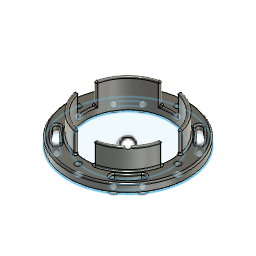
plunger holder v1 (Autodesk Fusion 360 design; units mm, degrees)
Autodesk Fusion 360 part; units mm, degrees
sketch "Sketch1" plane through (0, 0, 0) normal (0, 0, 1) x (1, 0, 0)
  circle A0 centre (-41.909966, 0.053051) radius 2.55
  circle A1 centre (41.91, 0) radius 2.55
  circle A2 centre (0, -41.910001) radius 2.55
  circle A3 centre (0, 41.910001) radius 2.55
  arc A4 (-25.400001, 38.100001) -> (-38.100001, 25.400001) centre (0, 0) ccw
  arc A5 (-38.100001, -25.400001) -> (-25.400001, -38.100001) centre (0, 0) ccw
  arc A6 (25.400001, -38.100001) -> (38.100001, -25.400001) centre (-1.334562, 1.334562) ccw
  arc A7 (38.100001, 25.400001) -> (25.400001, 38.100001) centre (-1.334562, -1.334562) ccw
  arc A8 (-22.582124, 33.873186) -> (-33.873186, 22.582124) centre (0, 0) ccw
  arc A9 (33.873186, 22.582124) -> (22.582124, 33.873186) centre (0, 0) ccw
  arc A10 (22.582124, -33.873186) -> (33.873186, -22.582124) centre (0, 0) ccw
  arc A11 (-33.873186, -22.582124) -> (-22.582124, -33.873186) centre (0, 0) ccw
  arc A12 (-33.873186, -22.582124) -> (-38.100001, -25.400001) centre (-35.986593, -23.991062) ccw
  arc A13 (-38.100001, 25.400001) -> (-33.873186, 22.582124) centre (-35.986593, 23.991062) ccw
  arc A14 (-22.582124, 33.873186) -> (-25.400001, 38.100001) centre (-23.991062, 35.986593) ccw
  arc A15 (25.400001, 38.100001) -> (22.582124, 33.873186) centre (23.991062, 35.986593) ccw
  arc A16 (33.873186, 22.582124) -> (38.100001, 25.400001) centre (35.986593, 23.991062) ccw
  arc A17 (38.100001, -25.400001) -> (33.873186, -22.582124) centre (35.99754, -23.974643) ccw
  arc A18 (22.582124, -33.873186) -> (25.400001, -38.100001) centre (23.974643, -35.99754) ccw
  arc A19 (-25.400001, -38.100001) -> (-22.582124, -33.873186) centre (-23.991062, -35.986593) ccw
  circle A20 centre (0, 0) radius 34.925
  circle A21 centre (0, 0) radius 50.165
  dimension "d4" = 5.1
  dimension "d5" = 5.1
  dimension "d6" = 5.1
  dimension "d7" = 5.1
  dimension "d24" = 69.85
  dimension "d25" = 100.33
  constraint tangent A5 A12
  constraint tangent A4 A13
  constraint tangent A8 A14
  constraint tangent A9 A15
  constraint tangent A9 A16
  constraint tangent A6 A17
  constraint tangent A6 A18
  constraint tangent A5 A19
  constraint concentric A10 A20
  measures "d4" diameter of A0
  measures "d5" diameter of A1
  measures "d6" diameter of A2
  measures "d7" diameter of A3
  measures "d24" diameter of A20
  measures "d25" diameter of A21
extrude "Extrude5" add sketch "Sketch1" along normal blind 7.62 contours A21 picked at (-41.009698, -9.190179)
sketch "Sketch3" plane through (0, 0, 7.62) normal (0, 0, 1) x (-1, 0, 0)
  arc A0 (-33.873186, -22.582124) -> (-38.100001, -25.400001) centre (-35.986593, -23.991062) ccw
  arc A1 (-33.873186, -22.582124) -> (-22.582124, -33.873186) centre (0, 0) ccw
  arc A2 (-25.400001, -38.100001) -> (-22.582124, -33.873186) centre (-23.991062, -35.986593) ccw
  arc A3 (-38.100001, -25.400001) -> (-25.400001, -38.100001) centre (1.334562, 1.334562) ccw
  circle A4 centre (-41.91, 0) radius 2.55
  circle A5 centre (0, 41.910001) radius 2.55
  arc A6 (-22.582124, 33.873186) -> (-25.400001, 38.100001) centre (-23.974643, 35.99754) ccw
  arc A7 (-22.582124, 33.873186) -> (-33.873186, 22.582124) centre (0, 0) ccw
  arc A8 (-38.100001, 25.400001) -> (-33.873186, 22.582124) centre (-35.99754, 23.974643) ccw
  arc A9 (-25.400001, 38.100001) -> (-38.100001, 25.400001) centre (1.334562, -1.334562) ccw
  arc A10 (22.582124, -33.873186) -> (25.400001, -38.100001) centre (23.991062, -35.986593) ccw
  arc A11 (22.582124, -33.873186) -> (33.873186, -22.582124) centre (0, 0) ccw
  arc A12 (38.100001, -25.400001) -> (33.873186, -22.582124) centre (35.986593, -23.991062) ccw
  arc A13 (25.400001, -38.100001) -> (38.100001, -25.400001) centre (0, 0) ccw
  circle A14 centre (41.909966, -0.053051) radius 2.55
  circle A15 centre (0, -41.910001) radius 2.55
  arc A16 (33.873186, 22.582124) -> (38.100001, 25.400001) centre (35.986593, 23.991062) ccw
  arc A17 (33.873186, 22.582124) -> (22.582124, 33.873186) centre (0, 0) ccw
  arc A18 (25.400001, 38.100001) -> (22.582124, 33.873186) centre (23.991062, 35.986593) ccw
  arc A19 (38.100001, 25.400001) -> (25.400001, 38.100001) centre (0, 0) ccw
  circle A20 centre (0, 0) radius 34.925
  circle A21 centre (0, 0) radius 50.165
  arc A22 (-8.470557, 33.882227) -> (-33.882227, 8.470557) centre (0, 0) ccw
  arc A23 (-9.086597, 36.346388) -> (-36.346388, 9.086597) centre (0, 0) ccw
  arc A24 (33.882227, 8.470557) -> (8.470557, 33.882227) centre (0, 0) ccw
  arc A25 (36.346388, 9.086597) -> (9.086597, 36.346388) centre (0, 0) ccw
  arc A26 (8.470557, -33.882227) -> (33.882227, -8.470557) centre (0, 0) ccw
  arc A27 (9.086597, -36.346388) -> (36.346388, -9.086597) centre (0, 0) ccw
  arc A28 (-33.882227, -8.470557) -> (-8.470557, -33.882227) centre (0, 0) ccw
  arc A29 (-36.346388, -9.086597) -> (-9.086597, -36.346388) centre (0, 0) ccw
  arc A30 (33.882227, 8.470557) -> (36.346388, 9.086597) centre (35.114308, 8.778577) ccw
  arc A31 (9.086597, 36.346388) -> (8.470557, 33.882227) centre (8.778577, 35.114308) ccw
  arc A32 (-8.470557, 33.882227) -> (-9.086597, 36.346388) centre (-8.778577, 35.114308) ccw
  arc A33 (-36.346388, 9.086597) -> (-33.882227, 8.470557) centre (-35.114308, 8.778577) ccw
  arc A34 (-33.882227, -8.470557) -> (-36.346388, -9.086597) centre (-35.114308, -8.778577) ccw
  arc A35 (-9.086597, -36.346388) -> (-8.470557, -33.882227) centre (-8.778577, -35.114308) ccw
  arc A36 (8.470557, -33.882227) -> (9.086597, -36.346388) centre (8.778577, -35.114308) ccw
  arc A37 (36.346388, -9.086597) -> (33.882227, -8.470557) centre (35.114308, -8.778577) ccw
  constraint tangent A25 A30
  constraint tangent A24 A31
  constraint tangent A23 A32
  constraint tangent A22 A33
  constraint tangent A28 A34
  constraint tangent A28 A35
  constraint tangent A26 A36
  constraint tangent A27 A37
extrude "Extrude6" add sketch "Sketch3" along normal blind 17.78 contours A20 A24 A25 A30 A31 | A20 A26 A27 A36 A37 | A20 A22 A23 A32 A33 | A20 A28 A29 A34 A35 picked at (35.006625, 10.485532) picked at (34.523393, -11.981049) picked at (-16.52197, 32.59501) picked at (-11.981049, -34.523393)
fillet "Fillet1" radius 1.27 16 edges at (26.491755, -26.491755, 25.4) (35.422328, -7.546496, 25.4) (24.695704, -24.695704, 25.4) (7.546496, -35.422328, 25.4) (-26.491755, -26.491755, 25.4) (-7.546496, -35.422328, 25.4) (-24.695704, -24.695704, 25.4) (-35.422328, -7.546496, 25.4) (26.491755, 26.491755, 25.4) (7.546496, 35.422328, 25.4) (24.695704, 24.695704, 25.4) (35.422328, 7.546496, 25.4) (-24.695704, 24.695704, 25.4) (-7.546496, 35.422328, 25.4) (-26.491755, 26.491755, 25.4) (-35.422328, 7.546496, 25.4)
fillet "Fillet4" radius 1.27 4 edges at (0, 34.925, 7.62) (34.925, 0, 7.62) (-34.925, 0, 7.62) (0, -34.925, 7.62)
fillet "Fillet5" radius 1.27 20 edges at (7.752154, 34.366403, 7.175515) (8.115639, 36.19755, 7.62) (26.491755, 26.491755, 7.62) (36.19755, 8.115639, 7.62) (34.366403, 7.752154, 7.175515) (-34.366403, 7.752154, 7.175515) (-36.19755, 8.115639, 7.62) (-26.491755, 26.491755, 7.62) (-8.115639, 36.19755, 7.62) (-7.752154, 34.366403, 7.175515) (-7.752154, -34.366403, 7.175515) (-8.115639, -36.19755, 7.62) (-26.491755, -26.491755, 7.62) (-36.19755, -8.115639, 7.62) (-34.366403, -7.752154, 7.175515) (34.366403, -7.752154, 7.175515) (36.19755, -8.115639, 7.62) (26.491755, -26.491755, 7.62) (8.115639, -36.19755, 7.62) (7.752154, -34.366403, 7.175515)
fillet "Fillet6" radius 1.27 2 edges at (-46.770201, -18.140438, 7.62) (-46.770201, -18.140438, 0)
fillet "Fillet7" radius 1.27 32 edges at (-21.877655, 37.395532, 7.62) (-28.786672, 28.786672, 7.62) (-37.395532, 21.877655, 7.62) (-32.378775, 32.378775, 7.62) (-21.877655, -37.395532, 7.62) (-32.378775, -32.378775, 7.62) (-37.395532, -21.877655, 7.62) (-28.786672, -28.786672, 7.62) (37.406521, -21.861171, 7.62) (32.353875, -32.353875, 7.62) (21.861171, -37.406521, 7.62) (28.786672, -28.786672, 7.62) (37.395532, 21.877655, 7.62) (28.786673, 28.786672, 7.62) (21.877655, 37.395532, 7.62) (32.353875, 32.353875, 7.62) (37.406521, -21.861171, 0) (32.353875, -32.353875, 0) (21.861171, -37.406521, 0) (37.395532, 21.877655, 0) (28.786673, 28.786672, 0) (21.877655, 37.395532, 0) (32.353875, 32.353875, 0) (-28.786672, 28.786672, 0) (-37.395532, 21.877655, 0) (-32.378775, 32.378775, 0) (-21.877655, 37.395532, 0) (-28.786672, -28.786672, 0) (-21.877655, -37.395532, 0) (-32.378775, -32.378775, 0) (-37.395532, -21.877655, 0) (28.786672, -28.786672, 0)
fillet "Fillet8" radius 1.27 1 edges at (-32.561533, 12.629419, 0)
